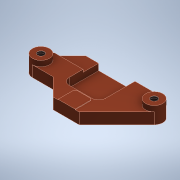
# Autodesk Inventor part: EPS_RegulatorHeatsink
Saved by Autodesk Inventor 2021 (Build 250183000, 183)
## iProperties
Created: 2020-12-05
Part Number: EPS_RegulatorHeatsink
Material: Copper
Document SubType Name: Modeling
Designer: Bradley
Density: 8.94 g/cm^3
Appearance: Copper - Satin
Author: Bradley
Autodesk Inventor part; units mm, degrees
ref_plane "YZ Plane" through (0, 0, 0) normal (1, 0, 0) x (0, 1, 0)
ref_plane "XZ Plane" through (0, 0, 0) normal (0, 1, 0) x (-1, 0, 0)
ref_plane "XY Plane" through (0, 0, 0) normal (0, 0, 1) x (1, 0, 0)
sketch "Sketch1" plane through (0, 0, 0) normal (0, 0, 1) x (1, 0, 0)
  line L0 (3.75, -3.75) -> (-3.75, -3.75) construction
  line L1 (-3.75, -3.75) -> (-3.75, 3.75) construction
  line L2 (-3.75, 3.75) -> (3.75, 3.75) construction
  line L3 (3.75, 3.75) -> (3.75, -3.75) construction
  line L4 (3.75, -3.75) -> (-3.75, 3.75) construction
  line L5 (-3.75, -3.75) -> (3.75, 3.75) construction
  line L6 (-6.9, -3.15) -> (-4.9, -3.15) construction
  line L7 (-4.9, -3.15) -> (-4.9, -1.15) construction
  line L8 (-4.9, -1.15) -> (-6.9, -1.15) construction
  line L9 (-6.9, -1.15) -> (-6.9, -3.15) construction
  line L10 (-6.9, -3.15) -> (-4.9, -1.15) construction
  line L11 (-4.9, -3.15) -> (-6.9, -1.15) construction
  line L12 (-0.5, -8) -> (2.5, -8) construction
  line L13 (2.5, -8) -> (2.5, -5) construction
  line L14 (2.5, -5) -> (-0.5, -5) construction
  line L15 (-0.5, -5) -> (-0.5, -8) construction
  line L16 (-0.5, -8) -> (2.5, -5) construction
  line L17 (2.5, -8) -> (-0.5, -5) construction
  circle A0 centre (-11.1, -2.4) radius 1.1
  circle A1 centre (-11.1, -2.4) radius 2
  circle A2 centre (11.3, 1.7) radius 1.1
  circle A3 centre (11.3, 1.7) radius 2
  line L18 (-2.1716, -8.5) -> (3.9284, -8.5)
  line L19 (3.9284, -8.5) -> (12.7142, 0.2858)
  line L20 (12.7142, 3.1142) -> (11.5784, 4.25)
  line L21 (11.5784, 4.25) -> (-7.2784, 4.25)
  line L22 (-7.2784, 4.25) -> (-12.5142, -0.9858)
  line L23 (-12, -7.9) -> (-9, -7.9) construction
  line L24 (-9, -7.9) -> (-9, -4.9) construction
  line L25 (-9, -4.9) -> (-12, -4.9) construction
  line L26 (-12, -4.9) -> (-12, -7.9) construction
  line L27 (-12, -7.9) -> (-9, -4.9) construction
  line L28 (-9, -7.9) -> (-12, -4.9) construction
  line L29 (-11.1, -4.4) -> (-6.2716, -4.4)
  line L30 (-6.2716, -4.4) -> (-2.1716, -8.5)
  line L31 (-4.25, 4.25) -> (-4.25, -2.65)
  arc A4 (-4.25, -2.65) -> (-2.65, -4.25) centre (-2.65, -2.65) ccw
  line L32 (-2.65, -4.25) -> (2.65, -4.25)
  arc A5 (2.65, -4.25) -> (4.25, -2.65) centre (2.65, -2.65) ccw
  line L33 (4.25, -2.65) -> (4.25, 4.25)
  line L34 (-10.9284, 0.6) -> (-4.25, 0.6)
  line L35 (3, -8.5) -> (3, -5)
  arc A6 (3, -5) -> (2.5, -4.5) centre (2.5, -5) ccw
  line L36 (-1, -8.5) -> (-1, -5)
  line L37 (2.5, -4.5) -> (-0.5, -4.5)
  arc A7 (-0.5, -4.5) -> (-1, -5) centre (-0.5, -5) ccw
  point P0 (0, 0)
  point P1 (-5.9, -2.15)
  point P2 (1, -6.5)
  point P3 (-10.5, -6.4)
  dimension "d0" = 6.5
  dimension "d1" = 1
  dimension "d2" = 5.9
  dimension "d3" = 2.15
  dimension "d4" = 7.5
  dimension "d5" = 3
  dimension "d6" = 2
  dimension "d7" = 2.2
  dimension "d8" = 4
  dimension "d9" = 11.1
  dimension "d10" = 2.4
  dimension "d11" = 11.3
  dimension "d12" = 1.7
  dimension "d16" = 0.5
  dimension "d17" = 0.5
  dimension "d20" = 10.5
  dimension "d21" = 6.4
  dimension "d22" = 3
  dimension "d23" = 135
  dimension "d24" = 1.6
  dimension "d25" = 0.5
  dimension "d28" = 3
  constraints: 78 end point, 13 perpendicular, 12 point on circle, 11 parallel, 11 tangent, 10 point on line, 8 centre point, 8 midpoint, 7 horizontal, 4 coincident, 3 equal radius, 2 vertical
  measures "d0" vertical distance of point (1, -6.5) point (0, 0)
  measures "d1" horizontal distance of point (1, -6.5) point (0, 0)
  measures "d2" horizontal distance of point (-5.9, -2.15) point (0, 0)
  measures "d3" vertical distance of point (-5.9, -2.15) point (0, 0)
  measures "d4" distance of L1.end L2.end
  measures "d5" distance of L13.end L14.end
  measures "d6" distance of L7.end L8.end
  measures "d7" diameter of A0
  measures "d8" diameter of A1
  measures "d9" horizontal distance of A0.centre point (0, 0)
  measures "d10" vertical distance of point (0, 0) A0.centre
  measures "d11" horizontal distance of A2.centre point (0, 0)
  measures "d12" vertical distance of point (0, 0) A2.centre
  measures "d16" distance between parallel lines of L2 L21
  measures "d17" distance between parallel lines of L18 L12
  measures "d20" horizontal distance of point (-10.5, -6.4) point (0, 0)
  measures "d21" vertical distance of point (-10.5, -6.4) point (0, 0)
  measures "d22" distance of L24.end L25.end
  measures "d23" angle of L18 L19
  measures "d24" radius of A4
  measures "d25" distance between parallel lines of L1 L31
  measures "d28" distance from line of A0.centre L34
extrude "Extrusion1" add sketch "Sketch1" against normal blind 3.9 contours A0 | A1 | A1 L22 L34 L31 A4 L32 A5 L33 L21 L20 A3 L19 L18 L35 A6 L37 A7 L36 L30 L29 | L22 L21 L31 L34 | L31 L21 L33 A5 L32 A4 | L36 A7 L37 A6 L35 L18 | A3 | A2
extrude "Extrusion2" cut sketch "Sketch1" against normal blind 3.4 contours L31 L21 L33 A5 L32 A4
extrude "Extrusion3" cut sketch "Sketch1" against normal blind 1.9 contours L22 L21 L31 L34
extrude "Extrusion4" cut sketch "Sketch1" against normal blind 1.3 contours A1 L22 L34 L31 A4 L32 A5 L33 L21 L20 A3 L19 L18 L35 A6 L37 A7 L36 L30 L29
extrude "Extrusion5" cut sketch "Sketch1" against normal blind 1.185 contours L36 A7 L37 A6 L35 L18
hole "Hole1" at (-11.1, -2.4, 0) at (11.3, 1.7, 0) direction (0, 0, -1) diameter 1.567 end through all thread size "M2x0.4" class "6H" standard "ANSI Metric M Profile"
equation "\"d17\" = d16"
body "Solid1"
